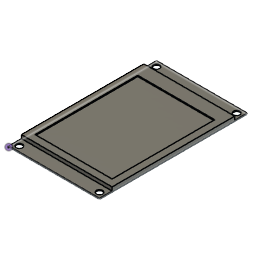
2.4 inch LCD display model (Autodesk Fusion 360 design; units mm, degrees)
part number: 2026-07-24-14-02-43-553
Autodesk Fusion 360 part; units mm, degrees
sketch "Sketch1" plane through (0, 0, 0) normal (0, 1, 0) x (1, 0, 0)
  line L0 (0, 0) -> (43.3, 0)
  line L1 (43.3, 0) -> (43.3, 70.5)
  line L2 (43.3, 70.5) -> (0, 70.5)
  line L3 (0, 70.5) -> (0, 0)
  dimension "d1" = 43.3
  dimension "d2" = 70.5
  constraint horizontal L0
  constraint vertical L1
  constraint horizontal L2
  constraint vertical L3
  constraint coincident L0.start L3.end
  measures "d1" distance of L0.start L0.end
  measures "d2" distance of L0.start L2.end
extrude "Extrude1" add sketch "Sketch1" along normal blind 0.5
sketch "Sketch2" plane through (0, 0.5, 0) normal (0, 1, 0) x (-1, 0, 0)
  line L0 (0, -70.5) -> (0, 0)
  line L1 (0, 0) -> (-43.3, 0)
  line L2 (-43.3, 0) -> (-43.3, -70.5)
  line L3 (-43.3, -70.5) -> (0, -70.5) construction
  line L4 (-43.3, 0) -> (-43.3, -5) construction
  line L5 (-43.3, -70.5) -> (-43.3, -64.5) construction
  line L6 (-43.3, -64.5) -> (0, -64.5)
  line L7 (0, -64.5) -> (0, -6)
  line L8 (0, -6) -> (-43.3, -6)
  line L9 (-43.3, -6) -> (-43.3, -64.5)
  line L10 (0, -2.5) -> (-2.5, -2.5) construction
  line L11 (-43.3, -2.5) -> (-40.8, -2.5) construction
  circle A0 centre (-2.5, -68) radius 1.5
  circle A1 centre (-40.8, -68) radius 1.5
  circle A2 centre (-40.8, -2.5) radius 1.5
  circle A3 centre (-2.5, -2.5) radius 1.5
  dimension "d5" = 6
  dimension "d8" = 2.5
  dimension "d10" = 3
  dimension "d11" = 3
  dimension "d12" = 3
  dimension "d13" = 3
  dimension "d16" = 2.5
  dimension "d17" = 2.5
  dimension "d18" = 2.5
  dimension "d19" = 2.5
  dimension "d20" = 2.5
  dimension "d21" = 2.5
  dimension "d22" = 2.5
  constraint coincident L1.end L2.start
  constraint coincident L2 L4.end
  constraint coincident L2.end L3.start
  constraint perpendicular L3 L5
  constraint horizontal L6
  constraint vertical L7
  constraint horizontal L8
  constraint vertical L9
  constraint coincident L0 L7.end
  constraint coincident L0 L10.start
  constraint perpendicular L0 L10
  constraint midpoint L4 L11.start
  constraint perpendicular L4 L11
  constraint coincident L11.end A2.centre
  constraint coincident L10.end A3.centre
  measures "d5" distance of L2.end L5.end
  measures "d8" distance of L11.start L11.end
  measures "d10" diameter of A0
  measures "d11" diameter of A1
  measures "d12" diameter of A2
  measures "d13" diameter of A3
  measures "d16" distance of L10.start L10.end
  measures "d17" distance of L1 L10.end
  measures "d18" distance of L1 L11.end
  measures "d19" distance of L5 A1.centre
  measures "d20" distance of L3 A1.centre
  measures "d21" distance of L3 A0.centre
  measures "d22" distance of L0 A0.centre
extrude "Extrude2" add sketch "Sketch2" along normal blind 1.67 contours L0 L2 L6 L7 L8 L9
extrude "Extrude3" cut sketch "Sketch2" against normal blind 5.737 contours A0 | A1 | A2 | A3
sketch "Sketch3" plane through (0, 2.17, 0) normal (0, 1, 0) x (-1, 0, 0)
  line L0 (-43.3, -6) -> (-43.3, -64.5)
  line L1 (-43.3, -64.5) -> (0, -64.5)
  line L2 (0, -64.5) -> (0, -6)
  line L3 (0, -6) -> (-43.3, -6)
  line L4 (-3.29, -9.29) -> (-40.01, -9.29)
  line L5 (-40.01, -9.29) -> (-40.01, -58.25)
  line L6 (-40.01, -58.25) -> (-3.29, -58.25)
  line L7 (-3.29, -58.25) -> (-3.29, -9.29)
  dimension "d23" = 36.72
  dimension "d24" = 48.96
  dimension "d25" = 3.29
  dimension "d26" = 3.29
  constraint horizontal L4
  constraint vertical L5
  constraint horizontal L6
  constraint vertical L7
  measures "d23" distance of L4.start L4.end
  measures "d24" distance of L4.start L6.end
  measures "d25" distance of L3 L4
  measures "d26" distance of L0 L5
extrude "Extrude4" cut sketch "Sketch3" against normal blind 0.5 contours L4 L5 L6 L7
